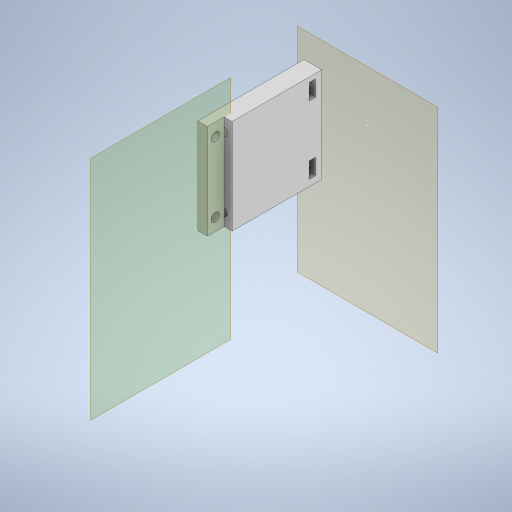
# Autodesk Inventor part: _108-64_adt
Saved by Autodesk Inventor 2024.3 (Build 283343000, 343)
## iProperties
Created: 2024-09-06
Part Number: _108-64_adt
Material: 일반
Document SubType Name: Modeling
Designer: gretc
Density: 1 g/cm^3
Appearance: 기본값
Author: gretc
Autodesk Inventor part; units mm, degrees
ref_plane "YZ Plane" through (0, 0, 0) normal (1, 0, 0) x (0, 1, 0)
ref_plane "XZ Plane" through (0, 0, 0) normal (0, 1, 0) x (-1, 0, 0)
ref_plane "XY Plane" through (0, 0, 0) normal (0, 0, 1) x (1, 0, 0)
ref_plane "작업 평면1" through (0, 0, 0) normal (0, 0, 1) x (1, 0, 0)
ref_plane "작업 평면2" through (-17, 0, 48.4) normal (-1, 0, 0) x (0, 0, 1)
sketch "스케치2" plane through (-17, 0, 48.4) normal (-1, 0, 0) x (0, 0, 1)
  line L0 (13.5, -39.75) -> (11.5, -39.75) projected
  arc A0 (11.5, -39.75) -> (9.25, -42) centre (11.5, -42) ccw projected
  line L1 (9.25, -42) -> (9.25, -44) projected
  arc A1 (8.25, -45) -> (9.25, -44) centre (8.25, -44) ccw projected
  line L2 (8.25, -45) -> (-8.25, -45) projected
  arc A2 (-9.25, -44) -> (-8.25, -45) centre (-8.25, -44) ccw projected
  line L3 (-9.25, -44) -> (-9.25, -42) projected
  arc A3 (-9.25, -42) -> (-11.5, -39.75) centre (-11.5, -42) ccw projected
  line L4 (-11.5, -39.75) -> (-13.5, -39.75) projected
  arc A4 (-14.5, -38.75) -> (-13.5, -39.75) centre (-13.5, -38.75) ccw projected
  line L5 (-14.5, -38.75) -> (-14.5, 8.25) projected
  arc A5 (-13.5, 9.25) -> (-14.5, 8.25) centre (-13.5, 8.25) ccw projected
  line L6 (-13.5, 9.25) -> (-11.5, 9.25) projected
  arc A6 (-11.5, 9.25) -> (-9.25, 11.5) centre (-11.5, 11.5) ccw projected
  line L7 (-9.25, 11.5) -> (-9.25, 14.5) projected
  line L8 (-15, 14.5) -> (-9.25, 14.5) projected
  line L9 (-20.1, 8.5) -> (-15, 14.5) projected
  line L10 (-20.1, -44.6) -> (-20.1, 8.5) projected
  line L11 (-15, -50.6) -> (-20.1, -44.6) projected
  line L12 (15, -50.6) -> (-15, -50.6) projected
  line L13 (20.1, -44.6) -> (15, -50.6) projected
  line L14 (20.1, 8.5) -> (20.1, -44.6) projected
  line L15 (15, 14.5) -> (20.1, 8.5) projected
  line L16 (9.25, 14.5) -> (15, 14.5) projected
  line L17 (9.25, 14.5) -> (9.25, 11.5) projected
  arc A7 (9.25, 11.5) -> (11.5, 9.25) centre (11.5, 11.5) ccw projected
  line L18 (11.5, 9.25) -> (13.5, 9.25) projected
  arc A8 (14.5, 8.25) -> (13.5, 9.25) centre (13.5, 8.25) ccw projected
  line L19 (14.5, 8.25) -> (14.5, -38.75) projected
  arc A9 (13.5, -39.75) -> (14.5, -38.75) centre (13.5, -38.75) ccw projected
  circle A10 centre (17.3, 4) radius 1.35 projected
  circle A11 centre (17.3, -18) radius 1.35 projected
  circle A12 centre (11, -47.8) radius 1.35 projected
  circle A13 centre (-17.3, 4) radius 1.35 projected
  circle A14 centre (-17.3, -18) radius 1.35 projected
  circle A15 centre (-11, -47.8) radius 1.35 projected
  circle A16 centre (17.3, -40) radius 1.35 projected
  circle A17 centre (-17.3, -40) radius 1.35 projected
  circle A18 centre (-17.3, -18) radius 2.8
  circle A19 centre (-17.3, 4) radius 2.8
  line L20 (-17.3, -18) -> (-17.3, 4)
  line L21 (-17.3, 4) -> (-17.3, -7)
  line L22 (-19.7531, 5.35) -> (-19.7531, -19.35)
  line L23 (-19.7531, -19.35) -> (-14.8469, -19.35)
  line L24 (-14.8469, -19.35) -> (-14.8469, 5.35)
  line L25 (-14.8469, 5.35) -> (-19.7531, 5.35)
  line L26 (-19.7531, 5.35) -> (-14.8469, -19.35) construction
  line L27 (-19.7531, -19.35) -> (-14.8469, 5.35) construction
  point P0 (-48.4, 0)
  point P1 (-19.7531, -19.35)
  point P2 (-14.8469, -19.35)
  point P3 (-14.8469, 5.35)
  point P4 (-19.7531, 5.35)
  dimension "d0" = 11
  constraints: 16 end point, 3 midpoint, 2 centre point, 2 coincident, 2 parallel, 2 tangent, 2 vertical, 1 perpendicular
  measures "d0" distance of L20.end L21.end
extrude "돌출1" add sketch "스케치2" along normal blind 3.1 contours A18 L23 | L23 A14 L20 A18 L24 | A18 L20 A19 L24 | L25 A19 | L24 A19 L20 A13 L25 | L22 A18 L20 A14 L23 | A18 L22 A19 L20 | L25 A13 L20 A19 L22
sketch "스케치3" plane through (-17, -19.35, 28.6469) normal (0, 0, -1) x (-1, 0, 0)
  line L0 (3.1, 24.7) -> (3.1, 0) projected
  line L1 (0, 0) -> (3.1, 0) projected
  line L2 (0, 24.7) -> (0, 0) projected
  line L3 (0, 0) -> (3.1, 0) projected
  line L4 (3.1, 24.7) -> (3.1, 0) projected
  line L5 (0, 24.7) -> (3.1, 24.7) projected
  point P0 (-17, 19.35)
extrude "돌출2" add sketch "스케치3" along normal blind 0.347
sketch "스케치4" plane through (-17, -19.35, 28.2999) normal (0, 0, -1) x (-1, 0, 0)
  line L0 (-4.5, 27.325) -> (-4.5, 25.825) projected
  line L1 (-4.5, 25.825) -> (-2.5, 25.825) projected
  line L2 (-2.5, 20.875) -> (-2.5, 25.825) projected
  line L3 (-4.5, 20.875) -> (-2.5, 20.875) projected
  line L4 (-4.5, 20.875) -> (-4.5, 19.375) projected
  line L5 (-4.5, 19.375) -> (-2, 19.375) projected
  line L6 (-2, 5.325) -> (-2, 19.375) projected
  line L7 (-2, 5.325) -> (-4.5, 5.325) projected
  line L8 (-4.5, 5.325) -> (-4.5, 3.825) projected
  line L9 (-4.5, 3.825) -> (-2.5, 3.825) projected
  line L10 (-2.5, -1.125) -> (-2.5, 3.825) projected
  line L11 (-4.5, -1.125) -> (-2.5, -1.125) projected
  line L12 (-4.5, -1.125) -> (-4.5, -2.625) projected
  line L13 (-4.5, -2.625) -> (-2, -2.625) projected
  line L14 (-2, -16.675) -> (-2, -2.625) projected
  line L15 (-2, -16.675) -> (-4.5, -16.675) projected
  line L16 (-4.5, -16.675) -> (-4.5, -18.175) projected
  line L17 (-4.5, -18.175) -> (-2.5, -18.175) projected
  line L18 (-2.5, -23.125) -> (-2.5, -18.175) projected
  line L19 (-4.5, -23.125) -> (-2.5, -23.125) projected
  line L20 (-4.5, -23.125) -> (-4.5, -24.625) projected
  line L21 (-4.5, -24.625) -> (-2, -24.625) projected
  line L22 (-2, -25.25) -> (-2, -24.625) projected
  line L23 (-2, -25.25) -> (0, -25.25) projected
  line L24 (0, -25.25) -> (0, 27.85) projected
  line L25 (-2, 27.85) -> (0, 27.85) projected
  line L26 (-2, 27.325) -> (-2, 27.85) projected
  line L27 (-2, 27.325) -> (-4.5, 27.325) projected
  line L28 (0, 0) -> (3.1, 0) projected
  line L29 (-2.5, 0) -> (0, 0)
  line L30 (3.1, 24.7) -> (0, 24.7) projected
  line L31 (-2.5, 24.7) -> (0, 24.7)
  line L32 (3.1, -2.625) -> (-2.5, -2.625) projected
  line L33 (-2.5, 27.325) -> (1.417, 27.325) projected
  line L34 (3.1, 24.7) -> (-2.5, 24.7)
  line L35 (-2.5, 24.7) -> (-2.5, 27.325)
  line L36 (-2.5, 27.325) -> (3.1, 27.325)
  line L37 (3.1, 27.325) -> (3.1, 24.7)
  line L38 (-2.5, 0) -> (3.1, 0)
  line L39 (3.1, 0) -> (3.1, -2.625)
  line L40 (3.1, -2.625) -> (-2.5, -2.625)
  line L41 (-2.5, -2.625) -> (-2.5, 0)
  line L42 (3.1, 23.9266) -> (3.1, -20.3266) projected
  line L43 (3.1, 0) -> (3.1, 24.7) projected
  circle A0 centre (0.3, 1.35) radius 1.35 projected
  circle A1 centre (0.3, 23.35) radius 1.35 projected
  point P0 (-17, 19.35)
  point P1 (1.417, 27.325)
  point P2 (-2.5, 25.825)
  point P3 (-2.5, -1.125)
  point P4 (-2.5, -2.625)
  point P5 (0.3, 24.7)
  point P6 (0, 24.6662)
  point P7 (0, 0.0338)
  point P8 (0.3, 0)
  constraints: 20 end point, 4 horizontal, 4 parallel, 2 perpendicular, 2 other
extrude "돌출3" add sketch "스케치4" along normal blind 28.3 contours L27 L33 L24 L31 L2 L35 | L31 L24 A1 A0 L29 L10 L9 L8 L7 L6 L5 L4 L3 L2 | L33 L36 L37 L30 L24 | L30 L43 L42 L28 A0 L24 A1 | L39 L32 L24 L28 | L24 L32 L13 L41 L10 L29
sketch "스케치6" plane through (-17, -19.35, -0.0001) normal (0, 0, -1) x (-1, 0, 0)
  point P0 (-17, 19.35)
sketch "스케치7" plane through (-20.1, 0, 48.4) normal (-1, 0, 0) x (0, 0, 1)
  line L0 (-20.1001, -15.525) -> (-48.4001, -15.525) projected
  line L1 (-20.1001, -19.35) -> (-48.4001, -19.35) projected
  line L2 (-48.4001, 2.65) -> (-20.1001, 2.65) projected
  line L3 (-20.1001, 5.35) -> (-48.4001, 5.35) projected
  line L4 (-48.4001, -19.35) -> (-45.4001, -19.35)
  line L5 (-45.4001, -19.35) -> (-45.4001, 5.35)
  line L6 (-43.3972, -19.35) -> (-43.3972, -17.4375)
  line L7 (-43.3972, -17.4375) -> (-45.4001, -17.4375)
  line L8 (-46.4001, -14.9375) -> (-46.4001, -19.9375)
  line L9 (-46.4001, -19.9375) -> (-44.4001, -19.9375)
  line L10 (-44.4001, -19.9375) -> (-44.4001, -14.9375)
  line L11 (-44.4001, -14.9375) -> (-46.4001, -14.9375)
  line L12 (-46.4001, -14.9375) -> (-44.4001, -19.9375) construction
  line L13 (-46.4001, -19.9375) -> (-44.4001, -14.9375) construction
  line L14 (-45.4001, 2.65) -> (-45.4001, 4)
  line L15 (-46.4001, 6.5) -> (-46.4001, 1.5)
  line L16 (-46.4001, 1.5) -> (-44.4001, 1.5)
  line L17 (-44.4001, 1.5) -> (-44.4001, 6.5)
  line L18 (-44.4001, 6.5) -> (-46.4001, 6.5)
  line L19 (-46.4001, 6.5) -> (-44.4001, 1.5) construction
  line L20 (-46.4001, 1.5) -> (-44.4001, 6.5) construction
  point P0 (-48.4, 0)
  dimension "d7" = 3
  dimension "d8" = 1.9125
  dimension "d9" = 2
  dimension "d10" = 1.35
  dimension "d11" = 5
  dimension "d12" = 5
  dimension "d13" = 2
  constraints: 34 end point, 7 point on line, 5 parallel, 4 midpoint, 4 perpendicular, 1 vertical
  measures "d7" distance of L1.end L4.end
  measures "d8" distance of L6.start L6.end
  measures "d9" distance of L9.end L8.end
  measures "d10" distance of L14.start L14.end
  measures "d11" distance between parallel lines of L11 L9
  measures "d12" distance of L15.start L15.end
  measures "d13" distance of L16.end L15.end
extrude "돌출4" cut sketch "스케치7" against normal blind 6 contours L10 L7 L5 L0 | L16 L15 L2 L5 | L5 L2 L17 L16 | L0 L5 L11 L10 | L5 L1 L8 L0 | L0 L8 L11 L5 | L10 L1 L5 L7 | L10 L9 L8 L1 | L5 L3 L17 L2 | L2 L15 L3 L5 | L15 L18 L17 L3
sketch "스케치8" plane through (-17, 0, 48.4) normal (-1, 0, 0) x (0, 0, 1)
  line L0 (-20.1001, -21.975) -> (-20.1001, -19.35) projected
  line L1 (-20.1001, -21.975) -> (-20.1001, 7.975)
  line L2 (-20.1001, 7.975) -> (-14.8422, 7.975)
  line L3 (-14.8422, 7.975) -> (-14.8422, -21.975)
  line L4 (-14.8422, -21.975) -> (-20.1001, -21.975)
  arc A0 (-19.7531, -19.35) -> (-14.8469, -19.35) centre (-17.3, -18) ccw projected
  line L5 (-19.7531, -19.35) -> (-20.1001, -19.35) projected
  line L6 (-20.1001, -19.3162) -> (-20.1001, -19.35) projected
  line L7 (-20.1001, -16.6838) -> (-20.1001, -19.3162) projected
  line L8 (-20.1001, 2.6838) -> (-20.1001, -16.6838) projected
  line L9 (-20.1001, 5.3162) -> (-20.1001, 2.6838) projected
  line L10 (-20.1001, 5.35) -> (-20.1001, 5.3162) projected
  line L11 (-19.7531, 5.35) -> (-20.1001, 5.35) projected
  arc A1 (-14.8469, 5.35) -> (-19.7531, 5.35) centre (-17.3, 4) ccw projected
  line L12 (-14.8469, -19.35) -> (-14.8469, 5.35) projected
  circle A2 centre (-17.3, 4) radius 1.35 projected
  circle A3 centre (-17.3, -18) radius 1.35 projected
  point P0 (-48.4, 0)
  point P1 (-20.1001, 5.35)
  point P2 (-20.1001, -19.35)
  constraints: 8 end point, 2 parallel, 1 perpendicular, 1 vertical
extrude "돌출5" add sketch "스케치8" along normal blind 3.1 contours L0 L5 A0 L12 A1 L11 L1 L2 L3 L4
sketch "스케치9" plane through (-12.5, 0.025, 28.2999) normal (1, 0, 0) x (0, 0, -1)
  line L0 (0, 1.5) -> (0, 0) projected
  line L1 (0, 0) -> (28.3, 0) projected
  line L2 (28.3, 1.5) -> (28.3, 0) projected
  line L3 (0, 1.5) -> (28.3, 1.5) projected
  line L4 (0, -14.05) -> (0, -15.55) projected
  line L5 (0, -15.55) -> (28.3, -15.55) projected
  line L6 (28.3, -14.05) -> (28.3, -15.55) projected
  line L7 (0, -14.05) -> (28.3, -14.05) projected
  point P0 (28.2999, -0.025)
extrude "돌출6" cut sketch "스케치9" against normal up to surface (2 mm away)
sketch "스케치10" plane through (-15, -14.025, 28.2999) normal (1, 0, 0) x (0, 0, -1)
  line L0 (0, 14.05) -> (0, 0) projected
  line L1 (0, 0) -> (28.3, 0) projected
  line L2 (28.3, 14.05) -> (28.3, 0) projected
  line L3 (0, 14.05) -> (28.3, 14.05) projected
  point P0 (28.2999, 14.025)
extrude "돌출7" add sketch "스케치10" along normal up to surface (0.5 mm away)
